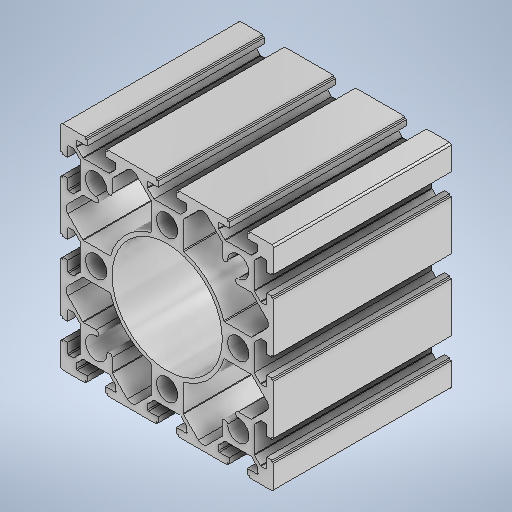
# Autodesk Inventor part: Perfil 120×120 12 rasgos_001
Saved by Autodesk Inventor 2026 (Build 300175000, 175)
## iProperties
Created: 2025-04-08
Part Number: Perfil 120×120 12 rasgos_001
Material: Aluminum 6061
Document SubType Name: Modeling
Designer: Tony Dias
Density: 2.7 g/cm^3
Appearance: Aluminum - Polished
Author: Tony Dias
Autodesk Inventor part; units mm, degrees
sketch "Sketch1" plane through (0, 0, 0) normal (0, 0, 1) x (1, 0, 0)
  circle A0 centre (0, 0) radius 31 construction
  circle A1 centre (-40, 40) radius 6 construction
  circle A2 centre (-40, 0) radius 6 construction
  line L0 (-49, 9) -> (-49, -9) construction
  line L1 (0, 0) -> (-60, 60) construction
  line L2 (-60, 20) -> (-40, 0) construction
  circle A3 centre (0, 0) radius 33.2 construction
  line L3 (-20, 20) -> (-40, 0) construction
  line L4 (-52.6556, 11.1) -> (-49, 7.4444)
  line L5 (-60, 5.1) -> (-56, 5.1) construction
  line L6 (-56, 5.1) -> (-56, 11.1)
  line L7 (-56, 11.1) -> (-52.6556, 11.1)
  line L8 (-60, 5.1) -> (-59, 5.1) construction
  line L9 (-59, 5.1) -> (-59, 6.1)
  line L10 (-59, 6.1) -> (-60, 6.1)
  line L11 (-60, 6.1) -> (-60, 5.1) construction
  line L12 (-59, 5.1) -> (-56, 5.1)
  line L13 (-60, 60) -> (-60, 45.1) construction
  line L14 (-49, 9) -> (-31.9568, 9) construction
  arc A4 (-23.4759, 23.4759) -> (-31.9568, 9) centre (0, 0) ccw
  line L15 (-49, 0) -> (-46, 0)
  line L16 (-49, 7.4444) -> (-49, 0)
  arc A5 (-34, 0) -> (-46, 0) centre (-40, 0) ccw
  line L17 (-34, 0) -> (-31, 0)
  line L18 (-56, 17.5556) -> (-47.4444, 9)
  line L19 (-47.4444, 9) -> (-31.9568, 9)
  line L20 (-40, 40) -> (-60, 20) construction
  line L21 (-49, 49) -> (-49, 31) construction
  line L22 (-49, 31) -> (-31, 31) construction
  line L23 (-47.4444, 31) -> (-56, 22.4444)
  arc A6 (-56, 22.4444) -> (-56, 17.5556) centre (-53.5556, 20) ccw
  line L24 (-49, 32.5556) -> (-52.6556, 28.9)
  line L25 (-52.6556, 28.9) -> (-56, 28.9)
  line L26 (-56, 28.9) -> (-56, 34.9)
  line L27 (-56, 34.9) -> (-60, 34.9) construction
  line L28 (-60, 34.9) -> (-59, 34.9) construction
  line L29 (-59, 34.9) -> (-59, 33.9)
  line L30 (-59, 33.9) -> (-60, 33.9)
  line L31 (-60, 33.9) -> (-60, 34.9) construction
  line L32 (-59, 34.9) -> (-56, 34.9)
  line L33 (-60, 33.9) -> (-60, 6.1)
  line L34 (-52.6556, 51.1) -> (-49, 47.4444)
  line L35 (-52.6556, 51.1) -> (-56, 51.1)
  line L36 (-56, 51.1) -> (-56, 45.1)
  line L37 (-56, 45.1) -> (-60, 45.1) construction
  line L38 (-60, 45.1) -> (-59, 45.1) construction
  line L39 (-59, 45.1) -> (-59, 46.1)
  line L40 (-59, 46.1) -> (-60, 46.1)
  line L41 (-60, 46.1) -> (-60, 45.1) construction
  line L42 (-59, 45.1) -> (-56, 45.1)
  line L43 (-60, 60) -> (-60, 46.1)
  line L44 (-47.4444, 31) -> (-40, 31)
  arc A7 (-44.2426, 44.2426) -> (-40, 34) centre (-40, 40) ccw
  arc A8 (-40, 31) -> (-40, 34) centre (-40, 32.5) ccw
  line L45 (-49, 47.4444) -> (-49, 32.5556)
  line L46 (-60, 60) -> (0, 0)
  arc A9 (-21.9203, 21.9203) -> (-31, 0) centre (0, 0) ccw
  point P0 (-32.5, 0)
  point P1 (-31, 0)
  dimension "d3" = 12
  dimension "d0" = 62
  dimension "d4" = 40
  dimension "d5" = 40
  dimension "d6" = 60
  dimension "d7" = 60
  dimension "d8" = 11
  dimension "d9" = 2.2
  dimension "d10" = 1.1
  dimension "d11" = 4
  dimension "d12" = 5.1
  dimension "d14" = 6
  dimension "d15" = 1
  dimension "d16" = 5.1
  dimension "d17" = 5.1
  dimension "d20" = 1.1
  dimension "d21" = 1.1
  dimension "d22" = 1.1
  dimension "d23" = 1.1
  constraints: 94 end point, 19 point on circle, 13 equal length, 13 point on line, 12 parallel, 10 horizontal, 9 centre point, 9 vertical alignment, 7 perpendicular, 5 coincident, 5 collinear, 4 horizontal alignment, 4 tangent, 4 vertical, 3 concentric, 3 midpoint, 4 other
  measures "d0" diameter of A0
  measures "d4" horizontal distance of point (0, 0) point (-40, 40)
  measures "d5" horizontal distance of point (0, 0) point (-40, 40)
  measures "d6" horizontal distance of point (0, 0) L1.end
  measures "d7" horizontal distance of point (0, 0) L1.end
  measures "d8" distance from line of L1.end L0
  measures "d9" radial gap between concentric circles of A0 A3
  measures "d10" distance between parallel lines of L2 L4
  measures "d11" distance of L5.start L5.end
  measures "d12" vertical distance of A2.centre L5.start
  measures "d14" distance of L5.end L6.end
  measures "d15" distance of L9.end L10.end
  measures "d16" vertical distance of point (-40, 40) L13.end
  measures "d17" vertical distance of point (-40, 40) L27.end
  measures "d20" distance between parallel lines of L2 L18
  measures "d21" distance between parallel lines of L20 L23
  measures "d22" distance between parallel lines of L20 L24
  measures "d23" distance between parallel lines of L1 L34
extrude "Extrusion1" add sketch "Sketch1" along normal mid plane 100 contours L7 L6 L12 L9 L10 L33 L30 L29 L32 L26 L25 L24 L45 L34 L35 L36 L42 L39 L40 L43 L46 A7 A8 L44 L23 A6 L18 L19 A4 A9 L17 A5 L15 L16 L4
fillet "Fillet2" radius 0.5 11 edges at (-56, 28.9, 0) (-52.6556, 28.9, 0) (-47.4444, 9, 0) (-52.6556, 11.1, 0) (-47.4444, 31, 0) (-52.6556, 51.1, 0) (-56, 51.1, 0) (-56, 11.1, 0) (-49, 32.5556, 0) (-49, 47.4444, 0) (-31.9568, 9, 0)
mirror "Mirror1" about plane through (-21.9203, 21.9203, 0) normal (0.7071068, 0.7071068, 0) of "Extrusion1", "Fillet2"
mirror "Mirror2" about plane through (0, 0, 0) normal (1, 0, 0) of "Extrusion1", "Fillet2", "Mirror1"
mirror "Mirror3" about plane through (0, 0, 0) normal (0, 1, 0) of "Extrusion1", "Fillet2", "Mirror1", "Mirror2"
fillet "Fillet3" radius 1 4 edges at (-60, 60, 0) (60, 60, 0) (60, -60, 0) (-60, -60, 0)
equation "\"d5\" = d4"
equation "\"d7\" = d6"
equation "\"d10\" = 0.5 * d9"
equation "\"d16\" = d12"
equation "\"d17\" = d12"
equation "\"d20\" = 0.5 * d9"
equation "\"d21\" = 0.5 * d9"
equation "\"d22\" = 0.5 * d9"
equation "\"d23\" = 0.5 * d9"
body "Solid1"
